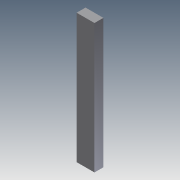
# Autodesk Inventor part: top-bot connector lame
Saved by Autodesk Inventor 2011 (Build 150239000, 239)
## iProperties
Created: 2011-08-20
Part Number: top-bot connector lame
Document SubType Name: Modeling
Designer: Matthew
Density: 1 g/cm^3
Author: Matthew
Autodesk Inventor part; units mm, degrees
ref_plane "YZ Plane" through (0, 0, 0) normal (1, 0, 0) x (0, 1, 0)
ref_plane "XZ Plane" through (0, 0, 0) normal (0, 1, 0) x (-1, 0, 0)
ref_plane "XY Plane" through (0, 0, 0) normal (0, 0, 1) x (1, 0, 0)
sketch "Sketch1" plane through (0, 0, 0) normal (0, 0, 1) x (1, 0, 0)
  line L0 (-22.2313, 26.7915) -> (109.8487, 26.7915)
  line L1 (109.8487, 26.7915) -> (109.8487, -144.6585)
  line L2 (109.8487, -144.6585) -> (-22.2313, -144.6585)
  line L3 (-22.2313, -144.6585) -> (-22.2313, 26.7915)
  line L4 (-22.2313, 26.7915) -> (-28.5813, 26.7915)
  line L5 (-28.5813, 26.7915) -> (-28.5813, 39.4915)
  line L6 (-28.5813, 39.4915) -> (116.1987, 39.4915)
  line L7 (116.1987, 39.4915) -> (116.1987, 26.7915)
  line L8 (116.1987, 26.7915) -> (128.8987, 26.7915)
  line L9 (128.8987, 26.7915) -> (128.8987, 14.0915)
  line L10 (128.8987, 14.0915) -> (116.1987, 14.0915)
  line L11 (116.1987, 14.0915) -> (116.1987, -131.9585)
  line L12 (116.1987, -131.9585) -> (128.8987, -131.9585)
  line L13 (128.8987, -131.9585) -> (128.8987, -144.6585)
  line L14 (128.8987, -144.6585) -> (116.1987, -144.6585)
  line L15 (116.1987, -144.6585) -> (116.1987, -154.1835)
  line L16 (116.1987, -154.1835) -> (-28.5813, -154.1835)
  line L17 (-28.5813, -154.1835) -> (-28.5813, -144.6585)
  line L18 (-28.5813, -144.6585) -> (-41.2813, -144.6585)
  line L19 (-41.2813, -144.6585) -> (-41.2813, -131.9585)
  line L20 (-41.2813, -131.9585) -> (-28.5813, -131.9585)
  line L21 (-28.5813, -131.9585) -> (-28.5813, 14.0915)
  line L22 (-28.5813, 14.0915) -> (-41.2813, 14.0915)
  line L23 (-41.2813, 14.0915) -> (-41.2813, 26.7915)
  line L24 (-41.2813, 26.7915) -> (-28.5813, 26.7915)
  line L25 (-22.2313, -144.6585) -> (-22.2313, -151.0085)
  line L26 (-22.2313, -151.0085) -> (15.8687, -151.0085)
  line L27 (15.8687, -151.0085) -> (15.8687, -144.6585)
  line L28 (15.8687, -144.6585) -> (22.2187, -144.6585)
  line L29 (22.2187, -144.6585) -> (22.2187, -151.0085)
  line L30 (109.8487, -144.6585) -> (109.8487, -151.0085)
  line L31 (109.8487, -151.0085) -> (71.7487, -151.0085)
  line L32 (71.7487, -151.0085) -> (71.7487, -144.6585)
  line L33 (71.7487, -144.6585) -> (65.3987, -144.6585)
  line L34 (65.3987, -144.6585) -> (65.3987, -151.0085)
  line L35 (65.3987, -151.0085) -> (22.2187, -151.0085)
  line L36 (-22.2313, 26.7915) -> (-22.2313, 33.1415)
  line L37 (-22.2313, 33.1415) -> (15.8687, 33.1415)
  line L38 (15.8687, 33.1415) -> (15.8687, 26.7915)
  line L39 (22.2187, 26.7915) -> (22.2187, 33.1415)
  line L40 (22.2187, 33.1415) -> (65.3987, 33.1415)
  line L41 (65.3987, 33.1415) -> (65.3987, 26.7915)
  line L42 (71.7487, 26.7915) -> (71.7487, 33.1415)
  line L43 (71.7487, 33.1415) -> (109.8487, 33.1415)
  line L44 (109.8487, 33.1415) -> (109.8487, 26.7915)
  circle A0 centre (-34.9313, 20.4415) radius 1.9812
  circle A1 centre (122.5487, 20.4415) radius 1.9812
  circle A2 centre (122.5487, -138.3085) radius 1.9812
  circle A3 centre (-34.9313, -138.3085) radius 1.9812
  point P0 (0, 0)
  dimension "d0" = 132.08
  dimension "d1" = 171.45
  dimension "d2" = 6.35
  dimension "d3" = 12.7
  dimension "d4" = 144.78
  dimension "d5" = 12.7
  dimension "d6" = 12.7
  dimension "d7" = 146.05
  dimension "d8" = 9.525
  dimension "d9" = 12.7
  dimension "d10" = 6.35
  dimension "d11" = 38.1
  dimension "d12" = 6.35
  dimension "d13" = 38.1
  dimension "d14" = 6.35
  dimension "d15" = 3.9624
  dimension "d16" = 3.9624
  constraints: 90 end point, 26 perpendicular, 16 parallel, 8 point on line, 4 centre point, 1 horizontal
  measures "d0" distance of L1.end L2.end
  measures "d1" distance of L0.end L1.end
  measures "d2" distance of L0.start L4.end
  measures "d3" distance of L4.end L5.end
  measures "d4" distance of L5.end L6.end
  measures "d5" distance of L7.end L8.end
  measures "d6" distance of L8.end L9.end
  measures "d7" distance of L10.end L11.end
  measures "d8" distance of L14.end L15.end
  measures "d9" distance of L17.end L18.end
  measures "d10" distance of L2.end L25.end
  measures "d11" distance of L25.end L26.end
  measures "d12" distance of L27.end L28.end
  measures "d13" distance of L30.end L31.end
  measures "d14" distance of L32.end L33.end
  measures "d15" diameter of A0
  measures "d16" diameter of A1
extrude "Extrusion1" add sketch "Sketch1" along normal blind 6.35
sketch "Sketch2" plane through (-28.5813, -154.1835, 0) normal (0, -1, 0) x (1, 0, 0)
  line L0 (144.78, 6.35) -> (0, 6.35) projected
  line L1 (0, 0) -> (0, 6.35) projected
  line L2 (0, 0) -> (144.78, 0) projected
  line L3 (144.78, 0) -> (144.78, 6.35) projected
  point P0 (28.5813, 0)
extrude "Extrusion2" add sketch "Sketch2" along normal blind 3.175
sketch "Sketch3" plane through (0, 0, 6.35) normal (0, 0, 1) x (1, 0, 0)
  line L0 (-28.5813, 14.0915) -> (-41.2813, 14.0915) projected
  line L1 (-28.5813, -131.9585) -> (-28.5813, 14.0915) projected
  line L2 (-41.2813, -131.9585) -> (-28.5813, -131.9585) projected
  line L3 (116.1987, -131.9585) -> (128.8987, -131.9585) projected
  line L4 (116.1987, 14.0915) -> (116.1987, -131.9585) projected
  line L5 (128.8987, 14.0915) -> (116.1987, 14.0915) projected
  line L6 (71.7487, 33.1415) -> (109.8487, 33.1415) projected
  line L7 (-41.2813, 14.0915) -> (-41.2813, -131.9585)
  line L8 (128.8987, 14.0915) -> (128.8987, -131.9585)
  point P0 (0, 0)
  constraints: 4 end point, 1 parallel, 1 perpendicular
extrude "Extrusion3" add sketch "Sketch3" against normal blind 6.35
sketch "Sketch4" plane through (0, 0, 6.35) normal (0, 0, 1) x (1, 0, 0)
  line L0 (-28.5813, -157.3585) -> (-28.5813, -144.6585) projected
  line L1 (-28.5813, -157.3585) -> (116.1987, -157.3585) projected
  line L2 (116.1987, -144.6585) -> (116.1987, -157.3585) projected
  line L3 (109.8487, 33.1415) -> (109.8487, -151.0085) projected
  line L4 (-22.2313, -151.0085) -> (-22.2313, 33.1415) projected
  line L5 (15.8687, 26.7915) -> (22.2187, 26.7915) projected
  line L6 (71.7487, 33.1415) -> (109.8487, 33.1415) projected
  line L7 (15.8687, 26.7915) -> (-22.2313, 26.7915)
  line L8 (22.2187, 26.7915) -> (109.8487, 26.7915)
  line L9 (109.8487, 26.7915) -> (109.8487, 20.4415)
  line L10 (109.8487, 20.4415) -> (-22.2313, 20.4415)
  line L11 (-22.2313, 20.4415) -> (-22.2313, 26.7915)
  line L12 (-22.2313, -144.6585) -> (-22.2313, -138.3085)
  line L13 (-22.2313, -138.3085) -> (109.8487, -138.3085)
  line L14 (109.8487, -144.6585) -> (-22.2313, -144.6585)
  line L15 (-28.5813, -151.0085) -> (-41.2813, -151.0085)
  line L16 (-41.2813, -151.0085) -> (-41.2813, -157.3585)
  line L17 (-41.2813, -157.3585) -> (-28.5813, -157.3585)
  line L18 (116.1987, -151.0085) -> (128.8987, -151.0085)
  line L19 (128.8987, -151.0085) -> (128.8987, -157.3585)
  line L20 (128.8987, -157.3585) -> (116.1987, -157.3585)
  point P0 (0, 0)
  constraints: 28 end point, 8 point on line, 6 perpendicular, 5 parallel, 2 midpoint, 1 collinear
extrude "Extrusion4" add sketch "Sketch4" against normal blind 6.35 contours L17 L16 L15 L0 | L2 L18 L19 L20 | L3 L10 L4 L7 L5 L8 | L3 L14 L4 L13
sketch "Sketch5" plane through (0, 0, 6.35) normal (0, 0, 1) x (1, 0, 0)
  line L0 (-28.5813, 26.7915) -> (-28.5813, 39.4915) projected
  line L1 (116.1987, 39.4915) -> (116.1987, 26.7915) projected
  line L2 (15.8687, 33.1415) -> (15.8687, 26.7915) projected
  line L3 (-28.5813, 39.4915) -> (-41.2813, 39.4915)
  line L4 (-41.2813, 39.4915) -> (-41.2813, 33.1415)
  line L5 (-41.2813, 33.1415) -> (-28.5813, 33.1415)
  line L6 (116.1987, 39.4915) -> (128.8987, 39.4915)
  line L7 (128.8987, 39.4915) -> (128.8987, 33.1415)
  line L8 (128.8987, 33.1415) -> (116.1987, 33.1415)
  point P0 (0, 0)
  constraints: 12 end point, 3 perpendicular, 2 midpoint, 1 parallel
extrude "Extrusion5" add sketch "Sketch5" against normal blind 6.35
sketch "Sketch6" plane through (0, 0, 6.35) normal (0, 0, 1) x (1, 0, 0)
  line L0 (65.3987, -151.0085) -> (22.2187, -151.0085) projected
  line L1 (22.2187, -144.6585) -> (65.3987, -144.6585) projected
  line L2 (-22.2313, -144.6585) -> (15.8687, -144.6585) projected
  line L3 (109.8487, -151.0085) -> (71.7487, -151.0085) projected
  line L4 (65.3987, 26.7915) -> (22.2187, 26.7915) projected
  line L5 (109.8487, 26.7915) -> (71.7487, 26.7915) projected
  line L6 (-41.2813, 26.7915) -> (-28.5813, 26.7915) projected
  line L7 (-28.5813, -151.0085) -> (-41.2813, -151.0085) projected
  line L8 (128.8987, -151.0085) -> (116.1987, -151.0085) projected
  line L9 (116.1987, 26.7915) -> (128.8987, 26.7915) projected
  line L10 (-28.5813, 33.1415) -> (-34.9313, 33.1415)
  line L11 (-34.9313, 33.1415) -> (-34.9313, 26.7915)
  line L12 (-34.9313, 26.7915) -> (-28.5813, 26.7915)
  line L13 (-28.5813, 26.7915) -> (-28.5813, 33.1415)
  line L14 (15.8687, 33.1415) -> (10.0792, 33.1415)
  line L15 (10.0792, 33.1415) -> (10.0792, 26.7915)
  line L16 (10.0792, 26.7915) -> (15.8687, 26.7915)
  line L17 (15.8687, 26.7915) -> (15.8687, 33.1415)
  line L18 (22.2187, 33.1415) -> (28.5687, 33.1415)
  line L19 (28.5687, 33.1415) -> (28.5687, 26.7915)
  line L20 (28.5687, 26.7915) -> (22.2187, 26.7915)
  line L21 (22.2187, 26.7915) -> (22.2187, 33.1415)
  line L22 (65.3987, 33.1415) -> (59.0487, 33.1415)
  line L23 (59.0487, 33.1415) -> (59.0487, 26.7915)
  line L24 (59.0487, 26.7915) -> (65.3987, 26.7915)
  line L25 (65.3987, 26.7915) -> (65.3987, 33.1415)
  line L26 (71.7487, 33.1415) -> (78.0987, 33.1415)
  line L27 (78.0987, 33.1415) -> (78.0987, 26.7915)
  line L28 (78.0987, 26.7915) -> (71.7487, 26.7915)
  line L29 (71.7487, 26.7915) -> (71.7487, 33.1415)
  line L30 (116.1987, 33.1415) -> (122.5487, 33.1415)
  line L31 (122.5487, 33.1415) -> (122.5487, 26.7915)
  line L32 (122.5487, 26.7915) -> (116.1987, 26.7915)
  line L33 (116.1987, 26.7915) -> (116.1987, 33.1415)
  line L34 (-28.5813, -144.6585) -> (-34.9313, -144.6585)
  line L35 (-34.9313, -144.6585) -> (-34.9313, -151.0085)
  line L36 (-34.9313, -151.0085) -> (-28.5813, -151.0085)
  line L37 (-28.5813, -151.0085) -> (-28.5813, -144.6585)
  line L38 (10.0792, -144.6585) -> (28.5687, -144.6585)
  line L39 (28.5687, -144.6585) -> (28.5687, -151.0085)
  line L40 (28.5687, -151.0085) -> (10.0792, -151.0085)
  line L41 (10.0792, -151.0085) -> (10.0792, -144.6585)
  line L42 (59.0487, -144.6585) -> (78.0987, -144.6585)
  line L43 (78.0987, -144.6585) -> (78.0987, -151.0085)
  line L44 (78.0987, -151.0085) -> (59.0487, -151.0085)
  line L45 (59.0487, -151.0085) -> (59.0487, -144.6585)
  line L46 (116.1987, -144.6585) -> (122.5487, -144.6585)
  line L47 (122.5487, -144.6585) -> (122.5487, -151.0085)
  line L48 (122.5487, -151.0085) -> (116.1987, -151.0085)
  line L49 (116.1987, -151.0085) -> (116.1987, -144.6585)
  point P0 (0, 0)
  dimension "d27" = 6.35
  dimension "d28" = 6.35
  dimension "d29" = 6.35
  dimension "d30" = 6.35
  dimension "d31" = 6.35
  constraints: 80 end point, 20 parallel, 10 horizontal, 10 perpendicular, 7 point on line, 4 midpoint
  measures "d27" distance of L15.end L14.end
  measures "d28" distance of L19.end L20.end
  measures "d29" distance of L24.end L23.end
  measures "d30" distance of L27.end L28.end
  measures "d31" distance of L31.end L32.end
extrude "Extrusion6" add sketch "Sketch6" against normal blind 6.35 contours L0 L45 L1 L42 L43 L3 L44 | L0 L40 L41 L2 L38 L1 L39 | L4 L21 L18 L19 | L4 L23 L22 L25 | L5 L29 L26 L27 | L11 L10 L13 L6 | L7 L35 L34 L37 | L8 L49 L46 L47 | L33 L30 L31 L9 | L17 L16 L15 L14
sketch "Sketch7" plane through (0, 0, 0) normal (0, 0, -1) x (-1, 0, 0)
  line L0 (-128.8987, 39.4915) -> (-90.7987, 39.4915)
  line L1 (-90.7987, 39.4915) -> (-90.7987, 115.6915)
  line L2 (-90.7987, 115.6915) -> (-128.8987, 115.6915)
  line L3 (-128.8987, 115.6915) -> (-128.8987, 39.4915)
  line L4 (-90.7987, 39.4915) -> (41.2813, 39.4915)
  line L5 (41.2813, 39.4915) -> (41.2813, 64.8915)
  line L6 (41.2813, 64.8915) -> (-90.7987, 64.8915)
  line L7 (-90.7987, 64.8915) -> (-90.7987, 39.4915)
  point P0 (0, 0)
  dimension "d34" = 38.1
  dimension "d35" = 76.2
  dimension "d36" = 25.4
  constraints: 16 end point, 4 parallel, 2 horizontal, 2 perpendicular
  measures "d34" distance of L2.end L1.end
  measures "d35" distance of L1.end L0.end
  measures "d36" distance of L5.end L4.end
extrude "Extrusion7" add sketch "Sketch7" against normal blind 6.35
sketch "Sketch8" plane through (0, 0, 0) normal (0, 0, -1) x (-1, 0, 0)
  line L0 (41.2813, 64.8915) -> (210.1913, 64.8915)
  line L1 (210.1913, 64.8915) -> (210.1913, 39.4915)
  line L2 (210.1913, 39.4915) -> (41.2813, 39.4915)
  line L3 (41.2813, 39.4915) -> (41.2813, 64.8915)
  line L4 (210.1913, 64.8915) -> (172.0913, 64.8915)
  line L5 (172.0913, 64.8915) -> (172.0913, 115.6915)
  line L6 (172.0913, 115.6915) -> (210.1913, 115.6915)
  line L7 (210.1913, 115.6915) -> (210.1913, 64.8915)
  point P0 (0, 0)
  dimension "d39" = 168.91
  dimension "d40" = 25.4
  dimension "d41" = 38.1
  constraints: 16 end point, 4 parallel, 2 horizontal, 2 perpendicular
  measures "d39" distance of L1.end L2.end
  measures "d40" distance of L0.end L1.end
  measures "d41" distance of L5.end L6.end
extrude "Extrusion8" add sketch "Sketch8" against normal blind 6.35
sketch "Sketch9" plane through (0, 0, 0) normal (0, 0, -1) x (-1, 0, 0)
  line L0 (-109.8487, 26.7915) -> (-109.8487, 33.1415) projected
  line L1 (-109.8487, 33.1415) -> (-78.0987, 33.1415) projected
  line L2 (-78.0987, 26.7915) -> (-78.0987, 33.1415) projected
  line L3 (-109.8487, 26.7915) -> (-78.0987, 26.7915) projected
  line L4 (-10.0792, 33.1415) -> (-10.0792, 26.7915) projected
  line L5 (-10.0792, 33.1415) -> (22.2313, 33.1415) projected
  line L6 (22.2313, 33.1415) -> (22.2313, 26.7915) projected
  line L7 (-10.0792, 26.7915) -> (22.2313, 26.7915) projected
  line L8 (-59.0487, 33.1415) -> (-28.5687, 33.1415) projected
  line L9 (-28.5687, 26.7915) -> (-28.5687, 33.1415) projected
  line L10 (-59.0487, 26.7915) -> (-28.5687, 26.7915) projected
  line L11 (-59.0487, 33.1415) -> (-59.0487, 26.7915) projected
  line L12 (-128.8987, 115.6915) -> (-128.8987, 33.1415) projected
  line L13 (-128.8987, 49.764) -> (41.2813, 49.764)
  line L14 (41.2813, 49.764) -> (41.2813, 26.7915)
  line L15 (41.2813, 26.7915) -> (-128.8987, 26.7915)
  line L16 (-128.8987, 26.7915) -> (-128.8987, 49.764)
  point P0 (0, 0)
  constraints: 8 end point, 2 parallel, 1 horizontal, 1 perpendicular, 1 point on line
extrude "Extrusion9" add sketch "Sketch9" against normal blind 6.35
sketch "Sketch10" plane through (0, 0, 0) normal (0, 0, -1) x (-1, 0, 0)
  line L0 (41.2813, 39.4915) -> (210.1913, 39.4915)
  line L1 (210.1913, 39.4915) -> (210.1913, 20.4415)
  line L2 (210.1913, 20.4415) -> (41.2813, 20.4415)
  line L3 (41.2813, 20.4415) -> (41.2813, 39.4915)
  point P0 (0, 0)
  constraints: 8 end point, 2 parallel, 1 horizontal, 1 perpendicular
extrude "Extrusion10" add sketch "Sketch10" against normal blind 6.35
sketch "Sketch11" plane through (0, 0, 0) normal (0, 0, -1) x (-1, 0, 0)
  line L0 (-128.8987, 115.6915) -> (-90.7987, 115.6915)
  line L1 (-90.7987, 115.6915) -> (-90.7987, 141.0915)
  line L2 (-90.7987, 141.0915) -> (-128.8987, 141.0915)
  line L3 (-128.8987, 141.0915) -> (-128.8987, 115.6915)
  line L4 (172.0913, 115.6915) -> (210.1913, 115.6915)
  line L5 (210.1913, 115.6915) -> (210.1913, 141.0915)
  line L6 (210.1913, 141.0915) -> (172.0913, 141.0915)
  line L7 (172.0913, 141.0915) -> (172.0913, 115.6915)
  point P0 (0, 0)
  dimension "d48" = 25.4
  constraints: 16 end point, 4 parallel, 2 horizontal, 2 perpendicular
  measures "d48" distance of L1.end L0.end
extrude "Extrusion11" add sketch "Sketch11" against normal blind 6.35
sketch "Sketch12" plane through (0, 0, 0) normal (0, 0, -1) x (-1, 0, 0)
  line L0 (210.1913, 20.4415) -> (172.0913, 20.4415)
  line L1 (172.0913, 20.4415) -> (172.0913, 26.7915)
  line L2 (172.0913, 26.7915) -> (210.1913, 26.7915)
  line L3 (210.1913, 26.7915) -> (210.1913, 20.4415)
  line L4 (172.0913, 26.7915) -> (146.6913, 26.7915)
  line L5 (146.6913, 26.7915) -> (146.6913, 33.1415)
  line L6 (146.6913, 33.1415) -> (172.0913, 33.1415)
  line L7 (172.0913, 33.1415) -> (172.0913, 26.7915)
  line L8 (146.6913, 33.1415) -> (172.0913, 33.1415)
  line L9 (172.0913, 33.1415) -> (172.0913, 39.4915)
  line L10 (172.0913, 39.4915) -> (146.6913, 39.4915)
  line L11 (146.6913, 39.4915) -> (146.6913, 33.1415)
  line L12 (146.6913, 39.4915) -> (95.8913, 39.4915)
  line L13 (95.8913, 39.4915) -> (95.8913, 33.1415)
  line L14 (95.8913, 33.1415) -> (146.6913, 33.1415)
  line L15 (146.6913, 33.1415) -> (146.6913, 39.4915)
  line L16 (95.8913, 39.4915) -> (70.4913, 39.4915)
  line L17 (70.4913, 39.4915) -> (70.4913, 33.1415)
  line L18 (70.4913, 33.1415) -> (95.8913, 33.1415)
  line L19 (95.8913, 33.1415) -> (95.8913, 39.4915)
  line L20 (146.6913, 33.1415) -> (133.9913, 33.1415)
  line L21 (133.9913, 33.1415) -> (133.9913, 26.7915)
  line L22 (133.9913, 26.7915) -> (146.6913, 26.7915)
  line L23 (146.6913, 26.7915) -> (146.6913, 33.1415)
  line L24 (133.9913, 33.1415) -> (108.5913, 33.1415)
  line L25 (108.5913, 33.1415) -> (108.5913, 26.7915)
  line L26 (108.5913, 26.7915) -> (133.9913, 26.7915)
  line L27 (133.9913, 26.7915) -> (133.9913, 33.1415)
  line L28 (70.4913, 33.1415) -> (57.7913, 33.1415)
  line L29 (57.7913, 33.1415) -> (57.7913, 26.7915)
  line L30 (57.7913, 26.7915) -> (70.4913, 26.7915)
  line L31 (70.4913, 26.7915) -> (70.4913, 33.1415)
  line L32 (57.7913, 26.7915) -> (32.3913, 26.7915)
  line L33 (32.3913, 26.7915) -> (32.3913, 33.1415)
  line L34 (32.3913, 33.1415) -> (57.7913, 33.1415)
  line L35 (57.7913, 33.1415) -> (57.7913, 26.7915)
  line L36 (32.3913, 33.1415) -> (19.6913, 33.1415)
  line L37 (19.6913, 33.1415) -> (19.6913, 26.7915)
  line L38 (19.6913, 26.7915) -> (32.3913, 26.7915)
  line L39 (32.3913, 26.7915) -> (32.3913, 33.1415)
  line L40 (19.6913, 33.1415) -> (-5.7087, 33.1415)
  line L41 (-5.7087, 33.1415) -> (-5.7087, 39.4915)
  line L42 (-5.7087, 39.4915) -> (19.6913, 39.4915)
  line L43 (19.6913, 39.4915) -> (19.6913, 33.1415)
  line L44 (-5.7087, 33.1415) -> (-18.4087, 33.1415)
  line L45 (-18.4087, 33.1415) -> (-18.4087, 26.7915)
  line L46 (-18.4087, 26.7915) -> (-5.7087, 26.7915)
  line L47 (-5.7087, 26.7915) -> (-5.7087, 33.1415)
  line L48 (-18.4087, 33.1415) -> (-43.8087, 33.1415)
  line L49 (-43.8087, 33.1415) -> (-43.8087, 26.7915)
  line L50 (-43.8087, 26.7915) -> (-18.4087, 26.7915)
  line L51 (-18.4087, 26.7915) -> (-18.4087, 33.1415)
  line L52 (-43.8087, 33.1415) -> (-56.5087, 33.1415)
  line L53 (-56.5087, 33.1415) -> (-56.5087, 26.7915)
  line L54 (-56.5087, 26.7915) -> (-43.8087, 26.7915)
  line L55 (-43.8087, 26.7915) -> (-43.8087, 33.1415)
  line L56 (-56.5087, 33.1415) -> (-81.9087, 33.1415)
  line L57 (-81.9087, 33.1415) -> (-81.9087, 38.8107)
  line L58 (-81.9087, 38.8107) -> (-56.5087, 38.8107)
  line L59 (-56.5087, 38.8107) -> (-56.5087, 33.1415)
  line L60 (-81.9087, 33.1415) -> (-94.6087, 33.1415)
  line L61 (-94.6087, 33.1415) -> (-94.6087, 26.7915)
  line L62 (-94.6087, 26.7915) -> (-81.9087, 26.7915)
  line L63 (-81.9087, 26.7915) -> (-81.9087, 33.1415)
  line L64 (-94.6087, 26.7915) -> (-120.0087, 26.7915)
  line L65 (-120.0087, 26.7915) -> (-120.0087, 33.1415)
  line L66 (-120.0087, 33.1415) -> (-94.6087, 33.1415)
  line L67 (-94.6087, 33.1415) -> (-94.6087, 26.7915)
  point P0 (0, 0)
  dimension "d51" = 6.35
  dimension "d52" = 25.4
  dimension "d53" = 6.35
  dimension "d54" = 25.4
  dimension "d55" = 6.35
  dimension "d56" = 50.8
  dimension "d57" = 25.4
  dimension "d58" = 12.7
  dimension "d59" = 25.4
  dimension "d60" = 12.7
  dimension "d61" = 25.4
  dimension "d62" = 12.7
  dimension "d63" = 25.4
  dimension "d64" = 12.7
  dimension "d65" = 25.4
  dimension "d66" = 12.7
  dimension "d67" = 25.4
  dimension "d68" = 12.7
  dimension "d69" = 25.4
  constraints: 136 end point, 34 parallel, 17 horizontal, 17 perpendicular, 1 point on line
  measures "d51" distance of L0.end L1.end
  measures "d52" distance of L5.end L6.end
  measures "d53" distance of L4.end L5.end
  measures "d54" distance of L10.end L9.end
  measures "d55" distance of L9.end L8.end
  measures "d56" distance of L14.end L13.end
  measures "d57" distance of L18.end L17.end
  measures "d58" distance of L22.end L21.end
  measures "d59" distance of L26.end L25.end
  measures "d60" distance of L30.end L29.end
  measures "d61" distance of L33.end L34.end
  measures "d62" distance of L38.end L37.end
  measures "d63" distance of L41.end L42.end
  measures "d64" distance of L46.end L45.end
  measures "d65" distance of L50.end L49.end
  measures "d66" distance of L54.end L53.end
  measures "d67" distance of L57.end L58.end
  measures "d68" distance of L62.end L61.end
  measures "d69" distance of L65.end L66.end
extrude "Extrusion12" cut sketch "Sketch12" against normal blind 6.35 contours L56 L57 L58 L59 | L40 L41 L42 L43 | L6 L11 L10 L9 | L26 L25 L14 L21 | L13 L18 L17 L16 | L29 L32 L33 L34 | L45 L50 L49 L48 | L61 L64 L65 L66
sketch "Sketch13" plane through (0, 0, 0) normal (0, 0, -1) x (-1, 0, 0)
  line L0 (210.1913, 20.4415) -> (210.1913, 141.0915) projected
  line L1 (210.1913, 20.4415) -> (203.8413, 20.4415)
  line L2 (203.8413, 20.4415) -> (203.8413, 64.8915)
  line L3 (203.8413, 64.8915) -> (210.1913, 64.8915)
  line L4 (210.1913, 64.8915) -> (210.1913, 20.4415)
  line L5 (203.8413, 64.8915) -> (210.1913, 64.8915)
  line L6 (210.1913, 64.8915) -> (210.1913, 90.2915)
  line L7 (210.1913, 90.2915) -> (203.8413, 90.2915)
  line L8 (203.8413, 90.2915) -> (203.8413, 64.8915)
  line L9 (203.8413, 90.2915) -> (210.1913, 90.2915)
  line L10 (210.1913, 90.2915) -> (210.1913, 115.6915)
  line L11 (210.1913, 115.6915) -> (203.8413, 115.6915)
  line L12 (203.8413, 115.6915) -> (203.8413, 90.2915)
  point P0 (0, 0)
  dimension "d72" = 6.35
  dimension "d73" = 25.4
  dimension "d74" = 25.4
  constraints: 24 end point, 6 parallel, 3 horizontal, 3 perpendicular, 2 point on line
  measures "d72" distance of L2.end L3.end
  measures "d73" distance of L6.end L5.end
  measures "d74" distance of L10.end L9.end
extrude "Extrusion13" cut sketch "Sketch13" against normal blind 6.35 contours L1 L2 L3 L0 | L7 L12 L11 L0
sketch "Sketch14" plane through (0, 0, 0) normal (0, 0, -1) x (-1, 0, 0)
  line L0 (-90.7987, 64.8915) -> (-90.7987, 141.0915) projected
  line L1 (-128.8987, -144.6585) -> (-128.8987, 141.0915) projected
  line L2 (-128.8987, 141.0915) -> (-90.7987, 141.0915)
  line L3 (-90.7987, 141.0915) -> (-90.7987, 115.6915)
  line L4 (-90.7987, 115.6915) -> (-128.8987, 115.6915)
  line L5 (-128.8987, 115.6915) -> (-128.8987, 141.0915)
  line L6 (172.0913, 141.0915) -> (210.1913, 141.0915)
  line L7 (210.1913, 141.0915) -> (210.1913, 115.6915)
  line L8 (210.1913, 115.6915) -> (172.0913, 115.6915)
  line L9 (172.0913, 115.6915) -> (172.0913, 141.0915)
  line L10 (-128.8987, 90.2915) -> (-122.5487, 90.2915)
  line L11 (-122.5487, 90.2915) -> (-122.5487, 64.8915)
  line L12 (-122.5487, 64.8915) -> (-128.8987, 64.8915)
  line L13 (-128.8987, 64.8915) -> (-128.8987, 90.2915)
  point P0 (0, 0)
  constraints: 24 end point, 6 parallel, 3 horizontal, 3 perpendicular, 2 point on line
extrude "Extrusion14" cut sketch "Sketch14" against normal blind 6.35
sketch "Sketch15" plane through (0, 0, 0) normal (0, 0, -1) x (-1, 0, 0)
  line L0 (203.8413, 20.4415) -> (203.8413, 64.8915) projected
  line L1 (203.8413, 39.4915) -> (197.4913, 39.4915)
  line L2 (197.4913, 39.4915) -> (197.4913, 26.7915)
  line L3 (197.4913, 26.7915) -> (203.8413, 26.7915)
  line L4 (203.8413, 26.7915) -> (203.8413, 39.4915)
  point P0 (0, 0)
  dimension "d79" = 6.35
  constraints: 8 end point, 2 parallel, 1 horizontal, 1 perpendicular, 1 point on line
  measures "d79" distance of L3.end L2.end
extrude "Extrusion15" cut sketch "Sketch15" against normal blind 6.35
sketch "Sketch16" plane through (0, 0, 0) normal (0, 0, -1) x (-1, 0, 0)
  line L0 (-128.8987, 90.2915) -> (-109.8487, 90.2915)
  line L1 (-109.8487, 90.2915) -> (-109.8487, 77.5915)
  line L2 (-109.8487, 77.5915) -> (-128.8987, 77.5915)
  line L3 (-128.8987, 77.5915) -> (-128.8987, 90.2915)
  line L4 (172.0913, 115.6915) -> (191.1413, 115.6915)
  line L5 (191.1413, 115.6915) -> (191.1413, 83.9415)
  line L6 (191.1413, 83.9415) -> (172.0913, 83.9415)
  line L7 (172.0913, 83.9415) -> (172.0913, 115.6915)
  circle A0 centre (-109.8487, 77.5915) radius 1.9812
  circle A1 centre (191.1413, 83.9415) radius 1.9812
  point P0 (0, 0)
  dimension "d82" = 19.05
  dimension "d83" = 3.9624
  dimension "d84" = 3.9624
  constraints: 16 end point, 4 parallel, 2 centre point, 2 coincident, 2 horizontal, 2 perpendicular
  measures "d82" distance of L5.end L6.end
  measures "d83" diameter of A0
  measures "d84" diameter of A1
extrude "Extrusion16" cut sketch "Sketch16" against normal blind 6.35 contours A0 L2 L1 | L1 L2 A0 | A1 L6 L5 | L5 L6 A1
sketch "Sketch17" plane through (0, 0, 0) normal (0, 0, -1) x (-1, 0, 0)
  line L0 (-122.5487, 90.2915) -> (-128.8987, 90.2915)
  line L1 (-128.8987, 90.2915) -> (-128.8987, 64.8915)
  line L2 (-128.8987, 64.8915) -> (-122.5487, 64.8915)
  line L3 (-122.5487, 64.8915) -> (-122.5487, 90.2915)
  point P0 (0, 0)
  constraints: 8 end point, 2 parallel, 1 horizontal, 1 perpendicular
extrude "Extrusion17" add sketch "Sketch17" against normal blind 6.35
sketch "Sketch18" plane through (0, 0, 0) normal (0, 0, -1) x (-1, 0, 0)
  line L0 (-128.8987, -144.6585) -> (-128.8987, 115.6915) projected
  line L1 (-128.8987, 115.6915) -> (-122.5487, 115.6915)
  line L2 (-122.5487, 115.6915) -> (-122.5487, 90.2915)
  line L3 (-122.5487, 90.2915) -> (-128.8987, 90.2915)
  line L4 (-128.8987, 90.2915) -> (-128.8987, 115.6915)
  line L5 (-128.8987, 90.2915) -> (-122.5487, 90.2915)
  line L6 (-122.5487, 90.2915) -> (-122.5487, 64.8915)
  line L7 (-122.5487, 64.8915) -> (-128.8987, 64.8915)
  line L8 (-128.8987, 64.8915) -> (-128.8987, 90.2915)
  line L9 (-122.5487, 64.8915) -> (-128.8987, 64.8915)
  line L10 (-128.8987, 64.8915) -> (-128.8987, 39.4915)
  line L11 (-128.8987, 39.4915) -> (-122.5487, 39.4915)
  line L12 (-122.5487, 39.4915) -> (-122.5487, 64.8915)
  point P0 (0, 0)
  dimension "d89" = 25.4
  dimension "d90" = 25.4
  dimension "d91" = 25.4
  constraints: 24 end point, 6 parallel, 3 horizontal, 3 perpendicular, 1 point on line
  measures "d89" distance of L1.end L2.end
  measures "d90" distance of L5.end L6.end
  measures "d91" distance of L10.end L9.end
extrude "Extrusion18" cut sketch "Sketch18" against normal blind 6.35 contours L0 L7 L12 L11 | L0 L1 L2 L3
sketch "Sketch19" plane through (0, 0, 0) normal (0, 0, -1) x (-1, 0, 0)
  line L0 (-122.5487, 90.2915) -> (-128.8987, 90.2915) projected
  line L1 (-128.8987, 64.8915) -> (-128.8987, 90.2915) projected
  line L2 (-128.8987, 64.8915) -> (-122.5487, 64.8915) projected
  line L3 (-122.5487, 64.8915) -> (-122.5487, 39.4915) projected
  line L4 (197.4913, 39.4915) -> (203.8413, 39.4915) projected
  line L5 (203.8413, 39.4915) -> (203.8413, 64.8915) projected
  line L6 (203.8413, 64.8915) -> (210.1913, 64.8915) projected
  line L7 (210.1913, 64.8915) -> (210.1913, 90.2915) projected
  line L8 (210.1913, 90.2915) -> (203.8413, 90.2915) projected
  line L9 (203.8413, 90.2915) -> (203.8413, 115.6915) projected
  line L10 (203.8413, 115.6915) -> (172.0913, 115.6915) projected
  line L11 (172.0913, 115.6915) -> (172.0913, 64.8915) projected
  line L12 (172.0913, 64.8915) -> (-90.7987, 64.8915) projected
  line L13 (-90.7987, 64.8915) -> (-90.7987, 115.6915) projected
  line L14 (-90.7987, 115.6915) -> (-122.5487, 115.6915) projected
  line L15 (-122.5487, 115.6915) -> (-122.5487, 90.2915) projected
  circle A0 centre (191.1413, 83.9415) radius 1.9812 projected
  circle A1 centre (-109.8487, 77.5915) radius 1.9812 projected
  line L16 (-81.9087, 38.8107) -> (-56.5087, 38.8107) projected
  line L17 (22.2313, 20.4415) -> (22.2313, -138.3085) projected
  line L18 (-122.5487, 39.4915) -> (197.4913, 39.4915)
  line L19 (-81.9087, 38.8107) -> (-81.9087, 39.4915)
  line L20 (-56.5087, 38.8107) -> (-56.5087, 39.4915)
  point P0 (0, 0)
  constraints: 6 end point, 2 perpendicular, 2 point on line, 1 parallel
extrude "Extrusion19" cut sketch "Sketch19" against normal blind 25.4
sketch "Sketch20" plane through (0, 0, 0) normal (0, 0, -1) x (-1, 0, 0)
  line L0 (32.3913, 33.1415) -> (57.7913, 33.1415) projected
  line L1 (57.7913, 33.1415) -> (57.7913, 26.7915) projected
  line L2 (57.7913, 26.7915) -> (32.3913, 26.7915) projected
  line L3 (32.3913, 26.7915) -> (32.3913, 33.1415) projected
  line L4 (-43.8087, 26.7915) -> (-43.8087, 33.1415) projected
  line L5 (-43.8087, 33.1415) -> (-18.4087, 33.1415) projected
  line L6 (-18.4087, 33.1415) -> (-18.4087, 26.7915) projected
  line L7 (-18.4087, 26.7915) -> (-43.8087, 26.7915) projected
  line L8 (108.5913, 26.7915) -> (108.5913, 33.1415) projected
  line L9 (108.5913, 33.1415) -> (133.9913, 33.1415) projected
  line L10 (133.9913, 33.1415) -> (133.9913, 26.7915) projected
  line L11 (133.9913, 26.7915) -> (108.5913, 26.7915) projected
  line L12 (-120.0087, 33.1415) -> (-94.6087, 33.1415) projected
  line L13 (-94.6087, 33.1415) -> (-94.6087, 26.7915) projected
  line L14 (-94.6087, 26.7915) -> (-120.0087, 26.7915) projected
  line L15 (-120.0087, 26.7915) -> (-120.0087, 33.1415) projected
  line L16 (-128.8987, 39.4915) -> (203.8413, 39.4915)
  line L17 (203.8413, 39.4915) -> (203.8413, 26.7915)
  line L18 (203.8413, 26.7915) -> (-128.8987, 26.7915)
  line L19 (-128.8987, 26.7915) -> (-128.8987, 39.4915)
  line L20 (203.8413, 26.7915) -> (41.2813, 26.7915)
  line L21 (41.2813, 26.7915) -> (41.2813, 20.4415)
  line L22 (41.2813, 20.4415) -> (203.8413, 20.4415)
  line L23 (203.8413, 20.4415) -> (203.8413, 26.7915)
  point P0 (0, 0)
  constraints: 16 end point, 4 parallel, 2 horizontal, 2 perpendicular
extrude "Extrusion20" cut sketch "Sketch20" against normal blind 25.4 contours L3 L18 L6 L5 L4 L13 L12 L15 L19 L16 L17 L10 L9 L8 L1 L0 | L0 L1 L2 L3 | L18 L11 L23 L22 L21 L2 | L7 L4 L5 L6 | L14 L15 L12 L13
sketch "Sketch21" plane through (0, 0, 6.35) normal (0, 0, 1) x (1, 0, 0)
  line L0 (128.8987, -157.3585) -> (128.8987, -151.0085) projected
  line L1 (128.8987, -151.0085) -> (122.5487, -151.0085) projected
  line L2 (122.5487, -151.0085) -> (122.5487, -144.6585) projected
  line L3 (128.8987, -144.6585) -> (122.5487, -144.6585) projected
  line L4 (128.8987, 26.7915) -> (128.8987, -144.6585) projected
  line L5 (128.8987, 26.7915) -> (-41.2813, 26.7915) projected
  line L6 (-22.2313, -138.3085) -> (-22.2313, 20.4415) projected
  line L7 (-22.2313, 20.4415) -> (109.8487, 20.4415) projected
  line L8 (109.8487, 20.4415) -> (109.8487, -138.3085) projected
  line L9 (109.8487, -138.3085) -> (-22.2313, -138.3085) projected
  line L10 (78.0987, -144.6585) -> (109.8487, -144.6585) projected
  line L11 (109.8487, -144.6585) -> (109.8487, -151.0085) projected
  line L12 (109.8487, -151.0085) -> (78.0987, -151.0085) projected
  line L13 (78.0987, -151.0085) -> (78.0987, -144.6585) projected
  circle A0 centre (122.5487, -138.3085) radius 1.9812 projected
  circle A1 centre (122.5487, 20.4415) radius 1.9812 projected
  line L14 (10.0792, -151.0085) -> (-22.2313, -151.0085) projected
  line L15 (-22.2313, -151.0085) -> (-22.2313, -144.6585) projected
  line L16 (-22.2313, -144.6585) -> (10.0792, -144.6585) projected
  line L17 (10.0792, -144.6585) -> (10.0792, -151.0085) projected
  line L18 (28.5687, -144.6585) -> (59.0487, -144.6585) projected
  line L19 (59.0487, -144.6585) -> (59.0487, -151.0085) projected
  line L20 (59.0487, -151.0085) -> (28.5687, -151.0085) projected
  line L21 (28.5687, -151.0085) -> (28.5687, -144.6585) projected
  line L22 (-22.2313, 26.7915) -> (128.8987, 26.7915)
  line L23 (128.8987, 26.7915) -> (128.8987, -157.3585)
  line L24 (128.8987, -157.3585) -> (-22.2313, -157.3585)
  line L25 (-22.2313, -157.3585) -> (-22.2313, 26.7915)
  line L26 (128.8987, -157.3585) -> (-41.2813, -157.3585)
  line L27 (-41.2813, -157.3585) -> (-41.2813, -144.6585)
  line L28 (-41.2813, -144.6585) -> (128.8987, -144.6585)
  line L29 (128.8987, -144.6585) -> (128.8987, -157.3585)
  point P0 (0, 0)
  constraints: 16 end point, 4 parallel, 2 horizontal, 2 perpendicular, 1 point on line
extrude "Extrusion21" cut sketch "Sketch21" against normal blind 25.4 contours L24 L25 L14 L17 L28 L21 L20 L19 L13 L12 L11 L2 L1 L0 | L1 L2 L3 L23 | L26 L27 L28 L15 L25 | L3 L28 L10 L18 L16 L25 L9 L8 L7 L5 L4 | L15 L16 L17 L14 | L11 L12 L13 L10 | L18 L19 L20 L21
sketch "Sketch22" plane through (0, 0, 6.35) normal (0, 0, 1) x (1, 0, 0)
  line L0 (-22.2313, -144.6585) -> (-22.2313, 26.7915) projected
  line L1 (-22.2313, 26.7915) -> (-41.2813, 26.7915) projected
  line L2 (-41.2813, 26.7915) -> (-41.2813, -144.6585) projected
  line L3 (-22.2313, -144.6585) -> (-41.2813, -144.6585) projected
  circle A0 centre (-34.9313, -138.3085) radius 1.9812 projected
  circle A1 centre (-34.9313, 20.4415) radius 1.9812 projected
  point P0 (0, 0)
extrude "Extrusion22" add sketch "Sketch22" against normal blind 12.7
sketch "Sketch23" plane through (0, 0, 6.35) normal (0, 0, 1) x (1, 0, 0)
  circle A0 centre (-34.9313, -138.3085) radius 1.9812 projected
  circle A1 centre (-34.9313, 20.4415) radius 1.9812 projected
  point P0 (0, 0)
extrude "Extrusion23" add sketch "Sketch23" against normal blind 12.7
sketch "Sketch24" plane through (0, 0, 6.35) normal (0, 0, 1) x (1, 0, 0)
  line L0 (-22.2313, -144.6585) -> (-41.2813, -144.6585) projected
  line L1 (-41.2813, 26.7915) -> (-34.9313, 26.7915)
  line L2 (-34.9313, 26.7915) -> (-34.9313, -144.6585)
  line L3 (-34.9313, -144.6585) -> (-41.2813, -144.6585)
  line L4 (-41.2813, -144.6585) -> (-41.2813, 26.7915)
  point P0 (0, 0)
  dimension "d104" = 6.35
  constraints: 8 end point, 2 parallel, 1 horizontal, 1 perpendicular, 1 point on line
  measures "d104" distance of L2.end L3.end
extrude "Extrusion24" cut sketch "Sketch24" against normal blind 12.7
sketch "Sketch25" plane through (-22.2313, 26.7915, 6.35) normal (0, 1, 0) x (1, 0, 0)
  line L0 (-12.7, 12.7) -> (-12.7, 0) projected
  line L1 (0, 0) -> (-12.7, 0) projected
  line L2 (0, 0) -> (0, 12.7) projected
  line L3 (0, 12.7) -> (-12.7, 12.7) projected
  point P0 (22.2313, 6.35)
extrude "Extrusion25" add sketch "Sketch25" along normal blind 12.7
sketch "Sketch26" plane through (-22.2313, -144.6585, -6.35) normal (0, -1, 0) x (1, 0, 0)
  line L0 (-12.7, 12.7) -> (-12.7, 0) projected
  line L1 (-12.7, 0) -> (0, 0) projected
  line L2 (0, 12.7) -> (0, 0) projected
  line L3 (0, 12.7) -> (-12.7, 12.7) projected
  point P0 (22.2313, 6.35)
extrude "Extrusion26" add sketch "Sketch26" along normal blind 6.35
sketch "Sketch27" plane through (-22.2313, 39.4915, 6.35) normal (1, 0, 0) x (0, 0, -1)
  line L0 (0, -190.5) -> (0, 0) projected
  line L1 (0, -190.5) -> (12.7, -190.5) projected
  line L2 (12.7, -190.5) -> (12.7, 0) projected
  line L3 (12.7, 0) -> (0, 0) projected
  point P0 (6.35, -39.4915)
extrude "Extrusion27" add sketch "Sketch27" along normal blind 6.35
sketch "Sketch28" plane through (0, 0, -6.35) normal (0, 0, -1) x (-1, 0, 0)
  line L0 (34.9313, -151.0085) -> (34.9313, 39.4915) projected
  line L1 (15.8813, 39.4915) -> (15.8813, -151.0085) projected
  line L2 (15.8813, -151.0085) -> (34.9313, -151.0085) projected
  line L3 (15.8813, -151.0085) -> (15.8813, -144.6585)
  line L4 (15.8813, -144.6585) -> (34.9313, -144.6585)
  point P0 (0, 0)
  dimension "d113" = 6.35
  constraints: 4 end point, 2 point on line, 1 perpendicular
  measures "d113" distance of L1.end L3.end
extrude "Extrusion28" cut sketch "Sketch28" against normal blind 12.7
sketch "Sketch29" plane through (-15.8813, 39.4915, 6.35) normal (1, 0, 0) x (0, 0, -1)
  line L0 (0, -184.15) -> (12.7, -184.15) projected
  line L1 (12.7, 0) -> (12.7, -184.15) projected
  line L2 (0, 0) -> (12.7, 0) projected
  line L3 (0, -184.15) -> (0, 0) projected
  point P0 (6.35, -39.4915)
extrude "Extrusion29" add sketch "Sketch29" along normal blind 6.35
sketch "Sketch30" plane through (-22.2313, 39.4915, 6.35) normal (0, 1, 0) x (1, 0, 0)
  line L0 (-12.7, 12.7) -> (12.7, 12.7) projected
  line L1 (-12.7, 0) -> (-12.7, 12.7) projected
  line L2 (12.7, 0) -> (-12.7, 0) projected
  line L3 (12.7, 0) -> (12.7, 12.7) projected
  point P0 (22.2313, 6.35)
extrude "Extrusion30" add sketch "Sketch30" along normal blind 12.7
sketch "Sketch31" plane through (-22.2313, 52.1915, 6.35) normal (0, 1, 0) x (1, 0, 0)
  line L0 (12.7, 12.7) -> (12.7, 0) projected
  line L1 (-12.7, 12.7) -> (12.7, 12.7) projected
  line L2 (-12.7, 0) -> (-12.7, 12.7) projected
  line L3 (12.7, 0) -> (-12.7, 0) projected
  point P0 (22.2313, 6.35)
extrude "Extrusion31" cut sketch "Sketch31" against normal blind 12.7
body "Solid1"
